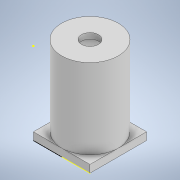
# Autodesk Inventor part: MotorSupport
Saved by Autodesk Inventor 2020.1 (Build 241239000, 239)
## iProperties
Created: 2019-11-07
Part Number: MotorSupport
Material: Generic
Document SubType Name: Modeling
Designer: super
Density: 1 g/cm^3
Appearance: Default
Author: super
Autodesk Inventor part; units mm, degrees
ref_plane "YZ Plane" through (0, 0, 0) normal (1, 0, 0) x (0, 1, 0)
ref_plane "XZ Plane" through (0, 0, 0) normal (0, 1, 0) x (-1, 0, 0)
ref_plane "XY Plane" through (0, 0, 0) normal (0, 0, 1) x (1, 0, 0)
sketch "Sketch1" plane through (0, 0, 0) normal (0, 1, 0) x (-1, 0, 0)
  line L0 (0, 0) -> (0, -45)
  line L1 (0, -45) -> (-45, -45)
  line L2 (-45, -45) -> (-45, 0)
  line L3 (-45, 0) -> (0, 0)
  dimension "d0" = 45
  dimension "d1" = 45
  dimension "d2" = 45
  constraints: 8 end point, 1 horizontal, 1 perpendicular, 1 vertical
  measures "d0" distance of L0.start L0.end
  measures "d1" distance of L0.end L1.end
  measures "d2" distance of L1.end L2.end
extrude "Extrusion1" add sketch "Sketch1" along normal blind 6
sketch "Sketch2" plane through (0, 6, 0) normal (0, 1, 0) x (1, 0, 0)
  line L0 (0, 0) -> (0, 22.5)
  line L1 (0, 45) -> (0, 0) projected
  line L2 (0, 22.5) -> (22.5, 22.5)
  circle A0 centre (22.5, 22.5) radius 22.5
  dimension "d5" = 22.5
  dimension "d6" = 22.5
  dimension "d7" = 45
  constraints: 4 end point, 1 centre point, 1 coincident, 1 midpoint, 1 perpendicular
  measures "d5" distance of L0.start L0.end
  measures "d6" distance of L0.end L2.end
  measures "d7" diameter of A0
extrude "Extrusion2" add sketch "Sketch2" along normal blind 63.5
sketch "Sketch3" plane through (0, 0, 0) normal (0, -1, 0) x (1, 0, 0)
  line L0 (0, -45) -> (0, 0) projected
  line L1 (0, 0) -> (0, -22.5)
  circle A0 centre (22.5, -22.5) radius 18.25
  dimension "d12" = 36.5
  constraints: 2 end point, 1 centre point, 1 midpoint
  measures "d12" diameter of A0
extrude "Extrusion3" cut sketch "Sketch3" against normal blind 65
sketch "Sketch4" plane through (22.5, 69.5, -22.5) normal (0, 1, 0) x (1, 0, 0)
  circle A0 centre (0, 0) radius 6.75
  point P0 (-22.5, -22.5)
  dimension "d15" = 13.5
  constraints: 1 centre point
  measures "d15" diameter of A0
extrude "Extrusion4" cut sketch "Sketch4" against normal blind 4.5
sketch "Sketch5" plane through (0, 0, 0) normal (0, -1, 0) x (1, 0, 0)
  line L0 (0, -45) -> (0, 0) projected
  line L1 (0, 0) -> (22.5, 0)
  line L2 (0, 0) -> (45, 0) projected
  constraints: 2 end point, 1 midpoint
sketch "Sketch6" plane through (22.5, 65, -22.5) normal (0, -1, 0) x (1, 0, 0)
  point P0 (-22.5, 22.5)
body "Solid1"
